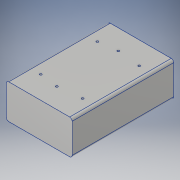
# Autodesk Inventor part: Elektronik_Gehäuse
Saved by Autodesk Inventor 2019 (Build 230136000, 136)
## iProperties
Created: 2018-04-27
Part Number: Elektronik_Gehäuse
Material: Aluminum 6061
Document SubType Name: Modeling
Designer: Phil Erle
Density: 2.7 g/cm^3
Appearance: Aluminum - Flat
Author: Phil Erle
Autodesk Inventor part; units mm, degrees
ref_plane "YZ Plane" through (0, 0, 0) normal (1, 0, 0) x (0, 1, 0)
ref_plane "XZ Plane" through (0, 0, 0) normal (0, 1, 0) x (-1, 0, 0)
ref_plane "XY Plane" through (0, 0, 0) normal (0, 0, 1) x (1, 0, 0)
sketch "Sketch1" plane through (0, 0, 0) normal (0, 0, 1) x (1, 0, 0)
  line L0 (-53.5, -82.5) -> (53.5, -82.5)
  line L1 (53.5, -82.5) -> (53.5, 82.5)
  line L2 (53.5, 82.5) -> (-53.5, 82.5)
  line L3 (-53.5, 82.5) -> (-53.5, -82.5)
  line L4 (-53.5, -82.5) -> (53.5, 82.5) construction
  line L5 (53.5, -82.5) -> (-53.5, 82.5) construction
  point P0 (0, 0)
  dimension "d0" = 107
  dimension "d1" = 165
  constraints: 12 end point, 2 midpoint, 2 parallel, 1 horizontal, 1 perpendicular
  measures "d0" distance of L1.end L2.end
  measures "d1" distance of L0.end L1.end
extrude "Extrusion1" add sketch "Sketch1" along normal blind 56
fillet "Fillet1" radius 4 4 edges at (-53.5, 0, 56) (53.5, 0, 56) (53.5, 0, 0) (-53.5, 0, 0)
sketch "Sketch2" plane through (0, 0, 56) normal (0, 0, 1) x (1, 0, 0)
  line L0 (-4, 50) -> (-4, -50) construction
  line L1 (-53.5, 82.5) -> (-53.5, -82.5) projected
  line L2 (53.5, -82.5) -> (53.5, 82.5) projected
  point P0 (0, 0)
  point P1 (-4, 0)
  dimension "d14" = 100
  dimension "d26" = 57.5
  constraints: 2 coincident, 2 end point, 1 horizontal alignment, 1 midpoint, 1 vertical
  measures "d14" distance of L0.start L0.end
  measures "d26" distance from line of L0.start L2
hole "Hole1" at (-4, -50, 56) at (-4, 50, 56) direction (0, 0, -1) diameter 3.4 depth 8 tip angle 118 clearance for "Countersunk Flat Head Screw DIN EN ISO 2009" size "M3" standard "DIN"
sketch "Sketch3" plane through (0, 0, 56) normal (0, 0, 1) x (1, 0, 0)
  line L0 (-34, -46) -> (34, -46) construction
  line L1 (34, -46) -> (34, 46) construction
  line L2 (34, 46) -> (-34, 46) construction
  line L3 (-34, 46) -> (-34, -46) construction
  line L4 (-49.5, -82.5) -> (49.5, -82.5) construction
  line L5 (-49.5, -82.5) -> (-49.5, 82.5) projected
  point P0 (0, 0)
  point P1 (0, -46)
  point P2 (-34, 0)
  point P3 (-49.5, 0)
  dimension "d16" = 92
  dimension "d17" = 68
  constraints: 8 end point, 4 coincident, 3 midpoint, 2 parallel, 1 horizontal, 1 horizontal alignment, 1 perpendicular, 1 vertical alignment
  measures "d16" distance of L2.end L0.start
  measures "d17" distance of L0.start L0.end
hole "Hole2" at (-34, -46, 56) at (-34, 46, 56) at (34, 46, 56) at (34, -46, 56) direction (0, 0, -1) diameter 3.4 depth 8 tip angle 118 clearance for "Countersunk Flat Head Screw DIN EN ISO 2009" size "M3" standard "DIN"
body "Solid1"
